Autodesk Fusion 360 part; units mm, degrees
(part 6 of 6)
  spline S241 degree 5 poles (-67.6889, 14.1982) (-67.6907, 14.1985) (-67.7009, 14.2008) (-67.7197, 14.2048) (-67.7471, 14.2106) (-67.783, 14.2181) (-67.8257, 14.2267) (-67.8685, 14.2351) (-67.9114, 14.2433) (-67.9544, 14.2513) (-67.9974, 14.2591) (-68.0406, 14.2667) (-68.0838, 14.2741) (-68.1271, 14.2814) (-68.1704, 14.2884) (-68.2138, 14.2952) (-68.2573, 14.3018) (-68.3009, 14.3083) (-68.3446, 14.3146) (-68.3883, 14.3207) (-68.432, 14.3266) (-68.4759, 14.3323) (-68.5198, 14.3378) (-68.5637, 14.3432) (-68.6078, 14.3484) (-68.6519, 14.3534) (-68.696, 14.3583) (-68.7402, 14.3629) (-68.7845, 14.3675) (-68.8288, 14.3718) (-68.8732, 14.376) (-68.9176, 14.38) (-68.9621, 14.3838) (-69.0067, 14.3875) (-69.0513, 14.391) (-69.0959, 14.3944) (-69.1406, 14.3976) (-69.1854, 14.4006) (-69.2302, 14.4035) (-69.275, 14.4062) (-69.32, 14.4088) (-69.3649, 14.4112) (-69.4099, 14.4134) (-69.455, 14.4155) (-69.5001, 14.4174) (-69.5452, 14.4192) (-69.5904, 14.4209) (-69.6266, 14.4221) (-69.6538, 14.4229) (-69.6719, 14.4234) (-69.6809, 14.4236) knots 0.354152 0.354152 0.354152 0.354152 0.354152 0.354152 0.357143 0.371429 0.385714 0.4 0.414286 0.428571 0.442857 0.457143 0.471429 0.485714 0.5 0.514286 0.528571 0.542857 0.557143 0.571429 0.585714 0.6 0.614286 0.628571 0.642857 0.657143 0.671429 0.685714 0.7 0.714286 0.728571 0.742857 0.757143 0.771429 0.785714 0.8 0.814286 0.828571 0.842857 0.857143 0.871429 0.885714 0.9 0.914286 0.928571 0.942857 0.957143 0.971429 0.985714 1 1 1 1 1 1
  arc A121 (-69.6809, 14.4236) -> (-69.985, 13.7803) centre (-40, 0) ccw
  spline S242 degree 5 poles (-69.985, 13.7803) (-69.9791, 13.7735) (-69.9672, 13.7598) (-69.9493, 13.7393) (-69.9254, 13.7121) (-69.8955, 13.6783) (-69.8654, 13.6445) (-69.8353, 13.6109) (-69.8051, 13.5774) (-69.7748, 13.5441) (-69.7444, 13.5108) (-69.7139, 13.4778) (-69.6833, 13.4448) (-69.6527, 13.412) (-69.6219, 13.3794) (-69.5911, 13.3468) (-69.5601, 13.3145) (-69.5291, 13.2822) (-69.498, 13.2501) (-69.4668, 13.2182) (-69.4355, 13.1864) (-69.4041, 13.1548) (-69.3726, 13.1233) (-69.341, 13.0919) (-69.3093, 13.0607) (-69.2776, 13.0297) (-69.2457, 12.9988) (-69.2138, 12.9681) (-69.1817, 12.9375) (-69.1495, 12.9071) (-69.1173, 12.8769) (-69.0849, 12.8468) (-69.0525, 12.8169) (-69.02, 12.7872) (-68.9873, 12.7576) (-68.9546, 12.7282) (-68.9217, 12.699) (-68.8888, 12.6699) (-68.8557, 12.641) (-68.8226, 12.6124) (-68.7893, 12.5839) (-68.756, 12.5555) (-68.7225, 12.5274) (-68.6889, 12.4995) (-68.6552, 12.4717) (-68.6215, 12.4442) (-68.5929, 12.4212) (-68.5711, 12.4037) (-68.556, 12.3918) (-68.5478, 12.3853) (-68.5464, 12.3841) knots -1 -1 -1 -1 -1 -1 -0.985714 -0.971429 -0.957143 -0.942857 -0.928571 -0.914286 -0.9 -0.885714 -0.871429 -0.857143 -0.842857 -0.828571 -0.814286 -0.8 -0.785714 -0.771429 -0.757143 -0.742857 -0.728571 -0.714286 -0.7 -0.685714 -0.671429 -0.657143 -0.642857 -0.628571 -0.614286 -0.6 -0.585714 -0.571429 -0.557143 -0.542857 -0.528571 -0.514286 -0.5 -0.485714 -0.471429 -0.457143 -0.442857 -0.428571 -0.414286 -0.4 -0.385714 -0.371429 -0.357143 -0.354152 -0.354152 -0.354152 -0.354152 -0.354152 -0.354152
  spline S243 degree 3 poles (-68.3949, 11.8001) (-68.3699, 11.8603) (-68.3569, 11.9247) (-68.3563, 12.0549) (-68.3688, 12.1194) (-68.4094, 12.2197) (-68.4307, 12.2574) (-68.4824, 12.3264) (-68.5126, 12.3574) (-68.5464, 12.3841) knots 0 0 0 0 0.019532 0.019532 0.039064 0.039064 0.051994 0.051994 0.064924 0.064924 0.064924 0.064924
  arc A122 (-68.3949, 11.8001) -> (-68.4273, 11.7219) centre (-40, 0) ccw
  spline S244 degree 3 poles (-68.9472, 11.4158) (-68.8825, 11.4083) (-68.817, 11.4135) (-68.6917, 11.4487) (-68.633, 11.4784) (-68.5478, 11.545) (-68.5174, 11.5758) (-68.4652, 11.6445) (-68.4437, 11.682) (-68.4273, 11.7219) knots 0 0 0 0 0.019532 0.019532 0.039064 0.039064 0.051994 0.051994 0.064924 0.064924 0.064924 0.064924
  spline S245 degree 5 poles (-68.9472, 11.4158) (-68.949, 11.416) (-68.9595, 11.4172) (-68.9786, 11.4194) (-69.0063, 11.4225) (-69.0428, 11.4264) (-69.0862, 11.4308) (-69.1296, 11.435) (-69.1731, 11.4389) (-69.2166, 11.4427) (-69.2603, 11.4462) (-69.3039, 11.4496) (-69.3476, 11.4527) (-69.3914, 11.4557) (-69.4353, 11.4584) (-69.4792, 11.4609) (-69.5231, 11.4633) (-69.5671, 11.4654) (-69.6111, 11.4674) (-69.6552, 11.4692) (-69.6994, 11.4707) (-69.7436, 11.4721) (-69.7878, 11.4734) (-69.8321, 11.4744) (-69.8764, 11.4753) (-69.9208, 11.4759) (-69.9652, 11.4764) (-70.0096, 11.4768) (-70.0541, 11.4769) (-70.0987, 11.4769) (-70.1432, 11.4767) (-70.1879, 11.4763) (-70.2325, 11.4758) (-70.2772, 11.4751) (-70.3219, 11.4742) (-70.3667, 11.4732) (-70.4115, 11.472) (-70.4564, 11.4706) (-70.5012, 11.4691) (-70.5461, 11.4674) (-70.5911, 11.4655) (-70.6361, 11.4635) (-70.6811, 11.4613) (-70.7261, 11.459) (-70.7712, 11.4565) (-70.8163, 11.4539) (-70.8614, 11.4511) (-70.8975, 11.4487) (-70.9247, 11.4469) (-70.9427, 11.4456) (-70.9518, 11.445) knots 0.354152 0.354152 0.354152 0.354152 0.354152 0.354152 0.357143 0.371429 0.385714 0.4 0.414286 0.428571 0.442857 0.457143 0.471429 0.485714 0.5 0.514286 0.528571 0.542857 0.557143 0.571429 0.585714 0.6 0.614286 0.628571 0.642857 0.657143 0.671429 0.685714 0.7 0.714286 0.728571 0.742857 0.757143 0.771429 0.785714 0.8 0.814286 0.828571 0.842857 0.857143 0.871429 0.885714 0.9 0.914286 0.928571 0.942857 0.957143 0.971429 0.985714 1 1 1 1 1 1
  arc A123 (-70.9518, 11.445) -> (-71.1914, 10.7749) centre (-40, 0) ccw
  spline S246 degree 5 poles (-71.1914, 10.7749) (-71.1848, 10.7687) (-71.1716, 10.7563) (-71.1518, 10.7376) (-71.1254, 10.7129) (-71.0922, 10.6821) (-71.059, 10.6515) (-71.0257, 10.621) (-70.9924, 10.5906) (-70.959, 10.5604) (-70.9255, 10.5303) (-70.8919, 10.5004) (-70.8582, 10.4706) (-70.8245, 10.441) (-70.7907, 10.4115) (-70.7568, 10.3821) (-70.7229, 10.353) (-70.6888, 10.3239) (-70.6547, 10.295) (-70.6205, 10.2663) (-70.5862, 10.2377) (-70.5519, 10.2093) (-70.5175, 10.1811) (-70.483, 10.153) (-70.4484, 10.125) (-70.4137, 10.0972) (-70.379, 10.0696) (-70.3442, 10.0422) (-70.3093, 10.0149) (-70.2743, 9.9878) (-70.2392, 9.9609) (-70.2041, 9.9341) (-70.1689, 9.9075) (-70.1336, 9.8811) (-70.0982, 9.8549) (-70.0627, 9.8288) (-70.0272, 9.803) (-69.9915, 9.7773) (-69.9558, 9.7518) (-69.92, 9.7265) (-69.8841, 9.7014) (-69.8482, 9.6765) (-69.8121, 9.6518) (-69.7759, 9.6273) (-69.7397, 9.603) (-69.7034, 9.5789) (-69.6727, 9.5588) (-69.6493, 9.5436) (-69.6331, 9.5331) (-69.6243, 9.5274) (-69.6228, 9.5265) knots -1 -1 -1 -1 -1 -1 -0.985714 -0.971429 -0.957143 -0.942857 -0.928571 -0.914286 -0.9 -0.885714 -0.871429 -0.857143 -0.842857 -0.828571 -0.814286 -0.8 -0.785714 -0.771429 -0.757143 -0.742857 -0.728571 -0.714286 -0.7 -0.685714 -0.671429 -0.657143 -0.642857 -0.628571 -0.614286 -0.6 -0.585714 -0.571429 -0.557143 -0.542857 -0.528571 -0.514286 -0.5 -0.485714 -0.471429 -0.457143 -0.442857 -0.428571 -0.414286 -0.4 -0.385714 -0.371429 -0.357143 -0.354152 -0.354152 -0.354152 -0.354152 -0.354152 -0.354152
  spline S247 degree 3 poles (-69.4148, 8.9601) (-69.3958, 9.0224) (-69.3892, 9.0878) (-69.4014, 9.2174) (-69.4201, 9.2805) (-69.4703, 9.3763) (-69.4952, 9.4117) (-69.5534, 9.4753) (-69.5865, 9.5032) (-69.6228, 9.5265) knots 0 0 0 0 0.019532 0.019532 0.039064 0.039064 0.051994 0.051994 0.064924 0.064924 0.064924 0.064924
  arc A124 (-69.4148, 8.9601) -> (-69.4394, 8.8791) centre (-40, 0) ccw
  spline S248 degree 3 poles (-69.9268, 8.5235) (-69.8617, 8.5224) (-69.797, 8.534) (-69.6757, 8.5813) (-69.6202, 8.6166) (-69.5419, 8.6912) (-69.5147, 8.7249) (-69.4695, 8.7983) (-69.4518, 8.8378) (-69.4394, 8.8791) knots 0 0 0 0 0.019532 0.019532 0.039064 0.039064 0.051994 0.051994 0.064924 0.064924 0.064924 0.064924
  spline S249 degree 5 poles (-69.9268, 8.5235) (-69.9286, 8.5235) (-69.9391, 8.5237) (-69.9583, 8.524) (-69.9863, 8.5244) (-70.0229, 8.5247) (-70.0665, 8.5248) (-70.1101, 8.5247) (-70.1538, 8.5244) (-70.1975, 8.5239) (-70.2413, 8.5231) (-70.2851, 8.5222) (-70.3289, 8.521) (-70.3728, 8.5196) (-70.4166, 8.5181) (-70.4606, 8.5163) (-70.5045, 8.5143) (-70.5485, 8.5121) (-70.5926, 8.5098) (-70.6366, 8.5072) (-70.6807, 8.5045) (-70.7248, 8.5015) (-70.7689, 8.4984) (-70.8131, 8.4951) (-70.8573, 8.4916) (-70.9015, 8.4879) (-70.9458, 8.4841) (-70.99, 8.48) (-71.0343, 8.4758) (-71.0787, 8.4714) (-71.123, 8.4669) (-71.1674, 8.4621) (-71.2118, 8.4572) (-71.2562, 8.4521) (-71.3006, 8.4469) (-71.3451, 8.4415) (-71.3895, 8.4359) (-71.434, 8.4301) (-71.4785, 8.4242) (-71.523, 8.4181) (-71.5676, 8.4119) (-71.6122, 8.4054) (-71.6567, 8.3989) (-71.7013, 8.3921) (-71.7459, 8.3852) (-71.7906, 8.3782) (-71.8352, 8.371) (-71.8709, 8.3651) (-71.8977, 8.3606) (-71.9156, 8.3576) (-71.9245, 8.356) knots 0.354152 0.354152 0.354152 0.354152 0.354152 0.354152 0.357143 0.371429 0.385714 0.4 0.414286 0.428571 0.442857 0.457143 0.471429 0.485714 0.5 0.514286 0.528571 0.542857 0.557143 0.571429 0.585714 0.6 0.614286 0.628571 0.642857 0.657143 0.671429 0.685714 0.7 0.714286 0.728571 0.742857 0.757143 0.771429 0.785714 0.8 0.814286 0.828571 0.842857 0.857143 0.871429 0.885714 0.9 0.914286 0.928571 0.942857 0.957143 0.971429 0.985714 1 1 1 1 1 1
  arc A125 (-71.9245, 8.356) -> (-72.0973, 7.6658) centre (-40, 0) ccw
  spline S250 degree 5 poles (-72.0973, 7.6658) (-72.0901, 7.6602) (-72.0758, 7.6491) (-72.0543, 7.6325) (-72.0255, 7.6105) (-71.9895, 7.5831) (-71.9535, 7.5559) (-71.9174, 7.5288) (-71.8812, 7.5018) (-71.845, 7.475) (-71.8087, 7.4484) (-71.7724, 7.4219) (-71.7359, 7.3956) (-71.6995, 7.3694) (-71.6629, 7.3433) (-71.6263, 7.3175) (-71.5897, 7.2917) (-71.553, 7.2662) (-71.5162, 7.2408) (-71.4793, 7.2155) (-71.4424, 7.1905) (-71.4055, 7.1655) (-71.3684, 7.1408) (-71.3314, 7.1162) (-71.2942, 7.0918) (-71.257, 7.0676) (-71.2197, 7.0435) (-71.1824, 7.0196) (-71.145, 6.9959) (-71.1075, 6.9723) (-71.07, 6.949) (-71.0324, 6.9258) (-70.9947, 6.9028) (-70.957, 6.8799) (-70.9192, 6.8573) (-70.8814, 6.8349) (-70.8434, 6.8126) (-70.8055, 6.7905) (-70.7674, 6.7687) (-70.7293, 6.747) (-70.6911, 6.7255) (-70.6529, 6.7043) (-70.6146, 6.6832) (-70.5762, 6.6624) (-70.5378, 6.6417) (-70.4992, 6.6213) (-70.4668, 6.6043) (-70.442, 6.5915) (-70.4249, 6.5827) (-70.4155, 6.5779) (-70.4139, 6.5771) knots -1 -1 -1 -1 -1 -1 -0.985714 -0.971429 -0.957143 -0.942857 -0.928571 -0.914286 -0.9 -0.885714 -0.871429 -0.857143 -0.842857 -0.828571 -0.814286 -0.8 -0.785714 -0.771429 -0.757143 -0.742857 -0.728571 -0.714286 -0.7 -0.685714 -0.671429 -0.657143 -0.642857 -0.628571 -0.614286 -0.6 -0.585714 -0.571429 -0.557143 -0.542857 -0.528571 -0.514286 -0.5 -0.485714 -0.471429 -0.457143 -0.442857 -0.428571 -0.414286 -0.4 -0.385714 -0.371429 -0.357143 -0.354152 -0.354152 -0.354152 -0.354152 -0.354152 -0.354152
  spline S251 degree 3 poles (-70.1514, 6.0338) (-70.1386, 6.0977) (-70.1384, 6.1634) (-70.1633, 6.2912) (-70.188, 6.3521) (-70.2475, 6.4425) (-70.2757, 6.4753) (-70.3399, 6.5329) (-70.3755, 6.5574) (-70.4139, 6.5771) knots 0 0 0 0 0.019532 0.019532 0.039064 0.039064 0.051994 0.051994 0.064924 0.064924 0.064924 0.064924
  arc A126 (-70.1514, 6.0338) -> (-70.1679, 5.9507) centre (-40, 0) ccw
  spline S252 degree 3 poles (-70.6181, 5.5491) (-70.5532, 5.5544) (-70.49, 5.5723) (-70.3739, 5.6312) (-70.3222, 5.6718) (-70.2515, 5.7538) (-70.2277, 5.7899) (-70.19, 5.8674) (-70.1762, 5.9085) (-70.1679, 5.9507) knots 0 0 0 0 0.019532 0.019532 0.039064 0.039064 0.051994 0.051994 0.064924 0.064924 0.064924 0.064924
  spline S253 degree 5 poles (-70.6181, 5.5491) (-70.6199, 5.549) (-70.6304, 5.5481) (-70.6496, 5.5465) (-70.6774, 5.5442) (-70.7139, 5.5409) (-70.7573, 5.5367) (-70.8007, 5.5323) (-70.8442, 5.5277) (-70.8876, 5.5229) (-70.9311, 5.5179) (-70.9746, 5.5127) (-71.0181, 5.5072) (-71.0616, 5.5015) (-71.1051, 5.4957) (-71.1486, 5.4896) (-71.1922, 5.4833) (-71.2358, 5.4769) (-71.2793, 5.4702) (-71.3229, 5.4633) (-71.3665, 5.4563) (-71.4102, 5.449) (-71.4538, 5.4416) (-71.4974, 5.434) (-71.541, 5.4262) (-71.5847, 5.4182) (-71.6283, 5.41) (-71.672, 5.4016) (-71.7157, 5.3931) (-71.7594, 5.3844) (-71.803, 5.3755) (-71.8467, 5.3664) (-71.8904, 5.3572) (-71.9341, 5.3478) (-71.9778, 5.3382) (-72.0215, 5.3285) (-72.0652, 5.3185) (-72.1089, 5.3084) (-72.1527, 5.2982) (-72.1964, 5.2878) (-72.2401, 5.2772) (-72.2838, 5.2664) (-72.3275, 5.2555) (-72.3713, 5.2444) (-72.415, 5.2332) (-72.4587, 5.2218) (-72.5024, 5.2103) (-72.5374, 5.2009) (-72.5636, 5.1938) (-72.5811, 5.189) (-72.5899, 5.1866) knots 0.354152 0.354152 0.354152 0.354152 0.354152 0.354152 0.357143 0.371429 0.385714 0.4 0.414286 0.428571 0.442857 0.457143 0.471429 0.485714 0.5 0.514286 0.528571 0.542857 0.557143 0.571429 0.585714 0.6 0.614286 0.628571 0.642857 0.657143 0.671429 0.685714 0.7 0.714286 0.728571 0.742857 0.757143 0.771429 0.785714 0.8 0.814286 0.828571 0.842857 0.857143 0.871429 0.885714 0.9 0.914286 0.928571 0.942857 0.957143 0.971429 0.985714 1 1 1 1 1 1
  arc A127 (-72.5899, 5.1866) -> (-72.6941, 4.4828) centre (-40, 0) ccw
  spline S254 degree 5 poles (-72.6941, 4.4828) (-72.6864, 4.4779) (-72.6711, 4.4683) (-72.648, 4.4539) (-72.6173, 4.4348) (-72.5788, 4.4111) (-72.5402, 4.3875) (-72.5016, 4.3641) (-72.463, 4.3408) (-72.4243, 4.3177) (-72.3856, 4.2947) (-72.3468, 4.2719) (-72.308, 4.2493) (-72.2692, 4.2268) (-72.2302, 4.2045) (-72.1913, 4.1823) (-72.1523, 4.1603) (-72.1132, 4.1385) (-72.0741, 4.1168) (-72.035, 4.0953) (-71.9958, 4.0739) (-71.9566, 4.0528) (-71.9173, 4.0318) (-71.878, 4.0109) (-71.8386, 3.9903) (-71.7992, 3.9698) (-71.7598, 3.9495) (-71.7203, 3.9294) (-71.6807, 3.9094) (-71.6411, 3.8897) (-71.6015, 3.8701) (-71.5618, 3.8507) (-71.5221, 3.8315) (-71.4823, 3.8125) (-71.4425, 3.7937) (-71.4026, 3.775) (-71.3627, 3.7566) (-71.3227, 3.7384) (-71.2827, 3.7203) (-71.2427, 3.7025) (-71.2026, 3.6849) (-71.1624, 3.6675) (-71.1222, 3.6503) (-71.082, 3.6333) (-71.0417, 3.6165) (-71.0014, 3.6) (-70.9674, 3.5862) (-70.9414, 3.5759) (-70.9236, 3.5688) (-70.9138, 3.565) (-70.9121, 3.5643) knots -1 -1 -1 -1 -1 -1 -0.985714 -0.971429 -0.957143 -0.942857 -0.928571 -0.914286 -0.9 -0.885714 -0.871429 -0.857143 -0.842857 -0.828571 -0.814286 -0.8 -0.785714 -0.771429 -0.757143 -0.742857 -0.728571 -0.714286 -0.7 -0.685714 -0.671429 -0.657143 -0.642857 -0.628571 -0.614286 -0.6 -0.585714 -0.571429 -0.557143 -0.542857 -0.528571 -0.514286 -0.5 -0.485714 -0.471429 -0.457143 -0.442857 -0.428571 -0.414286 -0.4 -0.385714 -0.371429 -0.357143 -0.354152 -0.354152 -0.354152 -0.354152 -0.354152 -0.354152
  spline S255 degree 3 poles (-70.5976, 3.0494) (-70.5912, 3.1142) (-70.5974, 3.1796) (-70.6347, 3.3044) (-70.6653, 3.3626) (-70.7333, 3.4467) (-70.7646, 3.4766) (-70.8341, 3.5276) (-70.872, 3.5485) (-70.9121, 3.5643) knots 0 0 0 0 0.019532 0.019532 0.039064 0.039064 0.051994 0.051994 0.064924 0.064924 0.064924 0.064924
  circle A128 centre (-40, 0) radius 25
  circle A129 centre (-40, 0) radius 28 construction
  circle A130 centre (-40, 0) radius 26.5
  line L0 (-40, 0) -> (-40, -55.0999) construction
  arc A131 (-44.8214, -26.566) -> (-35.1786, -26.566) centre (-40, 0) ccw
  arc A132 (-44.8214, -26.566) -> (-45.1786, -28.5339) centre (-45, -27.55) ccw
  arc A133 (-45.1786, -28.5339) -> (-34.8214, -28.5339) centre (-40, 0) ccw
  arc A134 (-34.8214, -28.5339) -> (-35.1786, -26.566) centre (-35, -27.55) ccw
  arc A135 (-45, -27.55) -> (-35, -27.55) centre (-40, 0) ccw construction
  arc A136 (-12.45, -5) -> (-12.45, 5) centre (-40, 0) ccw construction
  arc A137 (-13.434, -4.8214) -> (-13.434, 4.8214) centre (-40, 0) ccw
  arc A138 (-13.434, -4.8214) -> (-11.4661, -5.1786) centre (-12.45, -5) ccw
  arc A139 (-11.4661, 5.1786) -> (-13.434, 4.8214) centre (-12.45, 5) ccw
  arc A140 (-11.4661, -5.1786) -> (-11.4661, 5.1786) centre (-40, 0) ccw
  arc A141 (-35, 27.55) -> (-45, 27.55) centre (-40, 0) ccw construction
  arc A142 (-35.1786, 26.566) -> (-44.8214, 26.566) centre (-40, 0) ccw
  arc A143 (-35.1786, 26.566) -> (-34.8214, 28.5339) centre (-35, 27.55) ccw
  arc A144 (-45.1786, 28.5339) -> (-44.8214, 26.566) centre (-45, 27.55) ccw
  arc A145 (-34.8214, 28.5339) -> (-45.1786, 28.5339) centre (-40, 0) ccw
  arc A146 (-67.55, 5) -> (-67.55, -5) centre (-40, 0) ccw construction
  arc A147 (-66.566, 4.8214) -> (-66.566, -4.8214) centre (-40, 0) ccw
  arc A148 (-66.566, 4.8214) -> (-68.5339, 5.1786) centre (-67.55, 5) ccw
  arc A149 (-68.5339, -5.1786) -> (-66.566, -4.8214) centre (-67.55, -5) ccw
  arc A150 (-68.5339, 5.1786) -> (-68.5339, -5.1786) centre (-40, 0) ccw
  line L1 (-45, -27.55) -> (-35, -27.55) construction
  dimension "d31" = 56
  dimension "d32" = 1.5
  dimension "d33" = -1.5
  dimension "d38" = 360
  dimension "d43" = 10
  dimension "d44" = 1
  constraint concentric A0 A129
  constraint coincident A0.centre A1.centre
  constraint vertical L0
  constraint tangent A131 A132
  constraint tangent A132 A133
  constraint tangent A133 A134
  constraint tangent A131 A134
  constraint coincident A129 A132.centre
  constraint coincident A132.centre A135.start
  constraint coincident A134.centre A135.end
  constraint midpoint L0 L1
  measures "d31" diameter of A129
  measures "d43" distance of A134.centre A132.centre
  measures "d44" radius of A134
extrude "Extrude3" cut sketch "Sketch3 (3)" against normal blind 2 contours A131 A132 A133 A134 | A137 A138 A139 A140 | A142 A143 A144 A145 | A147 A148 A149 A150 sketch seen with x (0.998806, 0.04885, 0) y (-0.04885, 0.998806, 0) z (0, 0, 1) at (-39.9522, -1.954, 0) bodies 2 in component "Spur Gear (64 teeth)"
component "Spur Gear (16 teeth)" placed x (1, 0, 0) y (0, 1, 0) z (0, 0, 1) at (0, 0, 0)
component "Spur Gear (64 teeth)" placed x (0.998806, -0.04885, 0) y (0.04885, 0.998806, 0) z (0, 0, 1) at (40, 0, 0)
